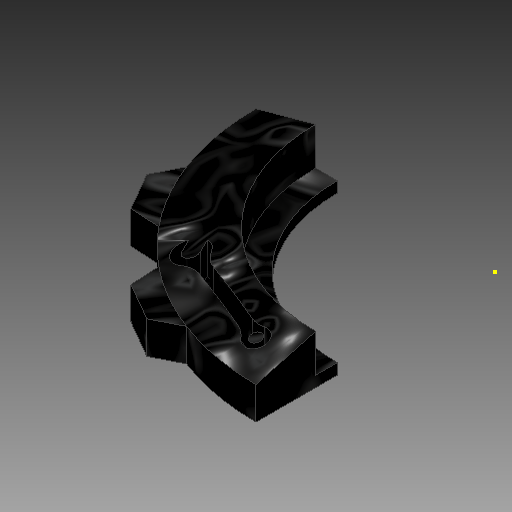
# Autodesk Inventor part: Mentor-Mechanical ring
Saved by Autodesk Inventor 2017 (Build 210142000, 142)
## iProperties
Created: 2016-02-20
Part Number: Mentor-Mechanical ring
Material: Generic
Document SubType Name: Modeling
Designer: RoksBot
Density: 1 g/cm^3
Appearance: Black
Author: RoksBot
Autodesk Inventor part; units mm, degrees
ref_plane "YZ Plane" through (0, 0, 0) normal (1, 0, 0) x (0, 1, 0)
ref_plane "XZ Plane" through (0, 0, 0) normal (0, 1, 0) x (-1, 0, 0)
sketch "Sketch1" plane through (0, 0, 0) normal (0, 0, 1) x (1, 0, 0)
  line L0 (0, 0) -> (0, 8.6646) construction
  line L1 (20.9931, 1.27) -> (20.9931, 5.715)
  line L2 (20.9931, 5.715) -> (27.9781, 3.81)
  line L3 (27.9781, 3.81) -> (27.9781, 0)
  line L4 (27.9781, 0) -> (20.9931, 0)
  line L5 (20.9931, 1.27) -> (18.4531, 1.27)
  line L6 (18.4531, 1.27) -> (18.4531, 0)
  line L7 (18.4531, 0) -> (20.9931, 0)
  dimension "d0" = 20.9931
  dimension "d1" = 4.445
  dimension "d2" = 1.27
  dimension "d3" = 2.54
  dimension "d4" = 3.81
  dimension "d5" = 6.985
  constraints: 16 end point, 2 parallel, 2 perpendicular, 2 vertical, 1 horizontal, 1 horizontal alignment
  measures "d0" distance between parallel lines of L0 L1
  measures "d1" distance from line of L5 L1.end
  measures "d2" distance of L5.end L6.end
  measures "d3" distance between parallel lines of L1 L6
  measures "d4" distance of L2.end L3.end
  measures "d5" distance between parallel lines of L1 L3
revolve "Revolution1" add sketch "Sketch1" angle 360 about axis through (0, 0, 0) along (0, 1, 0)
ref_plane "Work Plane1" through (0, 3.81, 0) normal (0, 1, 0) x (1, 0, 0)
sketch "Sketch2" plane through (0, 0, 0) normal (0, -1, 0) x (1, 0, 0)
  line L0 (0, 0) -> (-45.8206, 0) construction
  circle A0 centre (0, 0) radius 27.9781 projected
  line L1 (-27.6227, 4.445) -> (-30.5181, 2.54)
  line L2 (-30.5181, 2.54) -> (-30.5181, -2.54)
  line L3 (-30.5181, -2.54) -> (-27.6227, -4.445)
  dimension "d7" = 2.54
  dimension "d8" = 8.89
  dimension "d9" = 5.08
  constraints: 8 end point, 2 point on circle, 1 equal length, 1 horizontal, 1 vertical, 1 other
  measures "d7" distance edge to line of A0 L2
  measures "d8" distance of L3.end L1.start
  measures "d9" distance of L1.end L2.end
extrude "Extrusion1" add sketch "Sketch2" against normal up to surface (3.81 mm away) contours A0 L3 L2 L1
pattern_circular "Circular Pattern1" count 12 over 360 about axis through (0, 1.905, 0) along (0, -1, 0) of "Extrusion1"
sketch "Sketch4" plane through (0, 1.27, 0) normal (0, 1, 0) x (1, 0, 0)
  circle A0 centre (0, 0) radius 20.9931 projected
  arc A1 (-26.1445, 9.9619) -> (-27.6227, 4.445) centre (0, 0) ccw projected
  arc A2 (-27.6227, 4.445) -> (-27.6227, -4.445) centre (0, 0) ccw projected
  arc A3 (-27.6227, -4.445) -> (-26.1445, -9.9619) centre (0, 0) ccw projected
  arc A4 (-26.1445, -9.9619) -> (-21.6995, -17.6609) centre (0, 0) ccw projected
  arc A5 (-21.6995, -17.6609) -> (-17.6609, -21.6995) centre (0, 0) ccw projected
  arc A6 (-17.6609, -21.6995) -> (-9.9619, -26.1445) centre (0, 0) ccw projected
  arc A7 (-9.9619, -26.1445) -> (-4.445, -27.6227) centre (0, 0) ccw projected
  arc A8 (-4.445, -27.6227) -> (4.445, -27.6227) centre (0, 0) ccw projected
  arc A9 (4.445, -27.6227) -> (9.9619, -26.1445) centre (0, 0) ccw projected
  arc A10 (9.9619, -26.1445) -> (17.6609, -21.6995) centre (0, 0) ccw projected
  arc A11 (17.6609, -21.6995) -> (21.6995, -17.6609) centre (0, 0) ccw projected
  arc A12 (21.6995, -17.6609) -> (26.1445, -9.9619) centre (0, 0) ccw projected
  arc A13 (26.1445, -9.9619) -> (27.6227, -4.445) centre (0, 0) ccw projected
  arc A14 (27.6227, -4.445) -> (27.6227, 4.445) centre (0, 0) ccw projected
  arc A15 (27.6227, 4.445) -> (26.1445, 9.9619) centre (0, 0) ccw projected
  arc A16 (26.1445, 9.9619) -> (21.6995, 17.6609) centre (0, 0) ccw projected
  arc A17 (21.6995, 17.6609) -> (17.6609, 21.6995) centre (0, 0) ccw projected
  arc A18 (17.6609, 21.6995) -> (9.9619, 26.1445) centre (0, 0) ccw projected
  arc A19 (9.9619, 26.1445) -> (4.445, 27.6227) centre (0, 0) ccw projected
  arc A20 (4.445, 27.6227) -> (-4.445, 27.6227) centre (0, 0) ccw projected
  arc A21 (-4.445, 27.6227) -> (-9.9619, 26.1445) centre (0, 0) ccw projected
  arc A22 (-9.9619, 26.1445) -> (-17.6609, 21.6995) centre (0, 0) ccw projected
  arc A23 (-17.6609, 21.6995) -> (-21.6995, 17.6609) centre (0, 0) ccw projected
  arc A24 (-21.6995, 17.6609) -> (-26.1445, 9.9619) centre (0, 0) ccw projected
  circle A25 centre (0, 0) radius 18.4531 projected
  circle A26 centre (0, 0) radius 20.9931 projected
  circle A27 centre (24.1681, -3.81) radius 1.27
  circle A28 centre (24.1681, -3.81) radius 0.635
  line L0 (30.5181, 2.54) -> (30.5181, -2.54) projected
  arc A29 (17.9659, -17.8891) -> (17.3155, -16.3716) centre (19.0881, -16.51) ccw
  line L1 (19.0881, -16.51) -> (15.2571, -18.1519) construction
  line L2 (18.7629, -15.7512) -> (17.3155, -16.3716)
  line L3 (17.9659, -17.8891) -> (19.4133, -17.2688)
  arc A30 (19.4133, -17.2688) -> (18.7629, -15.7512) centre (19.0881, -16.51) ccw
  line L4 (19.0881, -16.51) -> (24.1681, -3.81) construction
  line L5 (19.1153, -14.7322) -> (23.17, -4.5954)
  line L6 (20.2945, -15.2039) -> (24.3492, -5.067)
  point P0 (17.1726, -17.3309)
  dimension "d19" = 2.54
  dimension "d20" = 0.635
  dimension "d22" = 3.81
  dimension "d23" = 6.35
  dimension "d24" = 3.556
  dimension "d25" = 135
  dimension "d26" = 1.27
  dimension "d27" = 0.635
  dimension "d28" = 12.7
  dimension "d29" = 5.08
  dimension "d30" = 1.651
  constraints: 14 end point, 8 point on circle, 4 centre point, 4 parallel, 2 tangent, 1 coincident, 1 midpoint
  measures "d19" diameter of A27
  measures "d20" radial gap between concentric circles of A27 A28
  measures "d22" vertical distance of A26.centre L4.end
  measures "d23" distance from line of L0 L4.end
  measures "d24" diameter of A29
  measures "d25" angle of L1 L4
  measures "d26" distance between parallel lines of L6 L5
  measures "d27" distance between parallel lines of L5 L4
  measures "d28" vertical distance of L1.start L4.end
  measures "d29" horizontal distance of A27.centre L1.start
  measures "d30" distance between parallel lines of L3 L2
extrude "Extrusion3" cut sketch "Sketch4" along normal through all contours A27 | A27 L6 A29 L5 | A29 L3 A30 L2
fillet "Fillet1" radius 3.175 4 edges at (19.1153, 3.0642, 14.7322) (20.2945, 2.8973, 15.2039) (23.17, 3.1341, 4.5954) (24.3492, 2.9637, 5.067)
pattern_circular "Circular Pattern2" count 3 over 90 about axis through (0, 3.4925, 0) along (0, -1, 0) of "Extrusion3", "Fillet1"
mirror "Mirror1" about plane through (0, 0, 0) normal (0, 0, 1) of "Extrusion3", "Fillet1", "Circular Pattern2"
sketch "Sketch5" plane through (0, 1.27, 0) normal (0, 1, 0) x (1, 0, 0)
  line L0 (0, 0) -> (-35.8156, 0)
  line L1 (-35.8156, 0) -> (-35.8156, -45.2748)
  line L2 (-35.8156, -45.2748) -> (0, -45.2748)
  line L3 (0, -45.2748) -> (0, 0)
  constraints: 8 end point, 2 parallel, 1 horizontal, 1 perpendicular
extrude "Extrusion4" cut sketch "Sketch5" along normal through all both and the other way through all keep common part
sketch "Sketch6" plane through (-2.54, 0, 30.5181) normal (0, -1, 0) x (1, 0, 0)
  line L0 (2.54, -9.525) -> (2.54, -2.54) projected
  arc A0 (2.54, -9.525) -> (-18.4531, -30.5181) centre (2.54, -30.5181) ccw projected
  line L1 (-25.4381, -30.5181) -> (-18.4531, -30.5181) projected
  arc A1 (-25.0827, -26.0731) -> (-25.4381, -30.5181) centre (2.54, -30.5181) ccw projected
  arc A2 (-23.6045, -20.5562) -> (-25.0827, -26.0731) centre (2.54, -30.5181) ccw projected
  arc A3 (-19.1595, -12.8572) -> (-23.6045, -20.5562) centre (2.54, -30.5181) ccw projected
  arc A4 (-15.1209, -8.8186) -> (-19.1595, -12.8572) centre (2.54, -30.5181) ccw projected
  arc A5 (-7.4219, -4.3736) -> (-15.1209, -8.8186) centre (2.54, -30.5181) ccw projected
  arc A6 (-1.905, -2.8954) -> (-7.4219, -4.3736) centre (2.54, -30.5181) ccw projected
  arc A7 (2.54, -2.54) -> (-1.905, -2.8954) centre (2.54, -30.5181) ccw projected
  line L2 (-3.6316, -6.6107) -> (-11.2674, -9.665) projected
  line L3 (-15.3491, -12.5522) -> (-14.7288, -11.1048) projected
  line L4 (-13.2112, -11.7552) -> (-13.8316, -13.2026) projected
  line L5 (-10.7957, -10.8442) -> (-3.1599, -7.7899) projected
  arc A8 (-23.6045, -20.5562) -> (-25.0827, -26.0731) centre (2.54, -30.5181) ccw projected
  line L6 (-25.0827, -26.0731) -> (-30.8234, -26.6683)
  line L7 (-30.8234, -26.6683) -> (-31.3133, -31.1273)
  line L8 (-31.3133, -31.1273) -> (-25.4381, -30.5181)
  line L9 (2.54, -2.54) -> (2.54, 0) projected
  arc A9 (2.54, -2.54) -> (-1.905, -2.8954) centre (2.54, -30.5181) ccw projected
  arc A10 (2.54, -2.54) -> (-1.905, -2.8954) centre (2.54, -30.5181) ccw
  line L10 (-1.905, -2.8954) -> (-3.1599, 4.5152)
  line L11 (-3.1599, 4.5152) -> (4.4262, 3.6816)
  line L12 (4.4262, 3.6816) -> (2.54, -2.54)
  point P0 (-2.2816, -5.5822)
  point P1 (-13.4231, -9.7382)
  point P2 (-12.4072, -12.2779)
  point P3 (-1.4731, -7.6037)
  constraints: 12 end point, 2 point on circle, 1 centre point, 1 parallel, 8 other
extrude "Extrusion5" cut sketch "Sketch6" along normal through all both and the other way through all contours A7 L10 L11 L12 | L8 L7 L6 A1
sketch "Sketch7" plane through (-20.9931, 1.27, 0) normal (0, 1, 0) x (1, 0, 0)
  point P0 (20.9931, 0)
equation "\"d27\" = 0.5 * d26"
body "Solid1"
